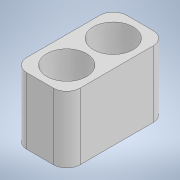
# Autodesk Inventor part: obudowa
Saved by Autodesk Inventor 2020.3 (Build 243373000, 373)
## iProperties
Created: 2021-04-25
Part Number: obudowa
Material: Ogólny
Document SubType Name: Modeling
Designer: patry
Density: 1 g/cm^3
Appearance: Domyślna
Author: patry
Autodesk Inventor part; units mm, degrees
ref_plane "YZ Plane" through (0, 0, 0) normal (1, 0, 0) x (0, 1, 0)
ref_plane "XZ Plane" through (0, 0, 0) normal (0, 1, 0) x (-1, 0, 0)
ref_plane "XY Plane" through (0, 0, 0) normal (0, 0, 1) x (1, 0, 0)
sketch "Szkic1" plane through (0, 0, 0) normal (0, 1, 0) x (-1, 0, 0)
  circle A0 centre (-0.3368, -8.6859) radius 3
  circle A1 centre (-0.3368, -1.6859) radius 3
  line L0 (3.6632, 2.3141) -> (-4.3368, 2.3141)
  line L1 (-4.3368, 2.3141) -> (-4.3368, -12.6859)
  line L2 (-4.3368, -12.6859) -> (3.6632, -12.6859)
  line L3 (3.6632, -12.6859) -> (3.6632, 2.3141)
  point P0 (0, 0)
  dimension "d0" = 6
  dimension "d1" = 6
  dimension "d2" = 7
  dimension "d3" = 8
  dimension "d4" = 15
  dimension "d5" = 4
  dimension "d6" = 4
  constraints: 8 end point, 2 centre point, 2 parallel, 1 horizontal, 1 perpendicular
  measures "d0" diameter of A0
  measures "d1" diameter of A1
  measures "d2" distance of A0.centre A1.centre
  measures "d3" distance of L2.end L1.end
  measures "d4" distance of L1.end L0.end
  measures "d5" distance from line of L3 A1.centre
  measures "d6" distance from line of L0 A1.centre
extrude "Wyciągnięcie proste1" add sketch "Szkic1" along normal blind 10
fillet "Zaokrąglenie1" radius 2 4 edges at (4.3368, 5, 2.3141) (-3.6632, 5, 2.3141) (4.3368, 5, -12.6859) (-3.6632, 5, -12.6859)
